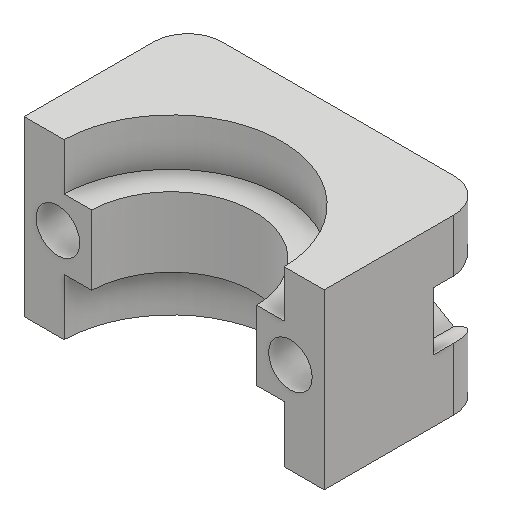
# Autodesk Inventor part: 3DP_ABS_E3DV6_Mounting_Clamp
Saved by Autodesk Inventor 2026.1 (Build 301233000, 233)
## iProperties
Created: 2016-01-19
Part Number: 3DP_ABS_E3DV6_Mounting_Clamp
Material: Ogólny
Document SubType Name: Modeling
Designer: Andrzej
Density: 1 g/cm^3
Appearance: Domyślna
Mass: 1.92147 g
Surface Area: 15.7734 cm^2
Volume: 1.92147 cm^3
Author: Andrzej
Autodesk Inventor part; units mm, degrees
ref_plane "YZ Plane" through (0, 0, 0) normal (1, 0, 0) x (0, 1, 0)
ref_plane "XZ Plane" through (0, 0, 0) normal (0, 1, 0) x (-1, 0, 0)
ref_plane "XY Plane" through (0, 0, 0) normal (0, 0, 1) x (1, 0, 0)
sketch "Szkic1" plane through (0, 0, 0) normal (0, 0, 1) x (1, 0, 0)
  line L0 (-13.054, 5.3954) -> (8.946, 5.3954)
  line L1 (8.946, 5.3954) -> (8.946, -6.6046)
  line L2 (8.946, -6.6046) -> (-13.054, -6.6046)
  line L3 (-13.054, -6.6046) -> (-13.054, 5.3954)
  point P0 (0, 0)
  dimension "d0" = 22
  dimension "d1" = 12
  constraints: 8 end point, 2 parallel, 1 horizontal, 1 perpendicular
  measures "d0" distance of L1.end L2.end
  measures "d1" distance of L0.end L1.end
extrude "Wyciągnięcie proste1" add sketch "Szkic1" along normal blind 12.7
fillet "Zaokrąglenie1" radius 2.5 2 edges at (-13.054, 5.3954, 6.35) (8.946, 5.3954, 6.35)
sketch "Szkic2" plane through (0, 0, 12.7) normal (0, 0, 1) x (1, 0, 0)
  line L0 (8.946, -6.6046) -> (8.946, 2.8954) projected
  line L1 (-13.054, 2.8954) -> (-13.054, -6.6046) projected
  circle A0 centre (-2.054, -6.8046) radius 8.075
  line L2 (6.446, 5.3954) -> (-10.554, 5.3954) projected
  point P0 (0, 0)
  dimension "d5" = 22
  dimension "d6" = 11
  dimension "d7" = 16.15
  dimension "d10" = 12.2
  constraints: 1 centre point, 1 coincident
  measures "d5" distance between parallel lines of L0 L1
  measures "d6" distance from line of L0 point (-2.054, -6.805)
  measures "d7" diameter of A0
  measures "d10" distance from line of L2 A0.centre
extrude "Wyciągnięcie proste2" cut sketch "Szkic2" against normal blind 12.7
sketch "Szkic3" plane through (0, 0, 12.7) normal (0, 0, 1) x (1, 0, 0)
  arc A0 (6.0185, -6.6046) -> (-10.1265, -6.6046) centre (-2.054, -6.8046) ccw projected
  line L0 (6.0185, -6.6046) -> (8.946, -6.6046) projected
  line L1 (8.946, -6.6046) -> (8.946, 2.8954) projected
  arc A1 (8.946, 2.8954) -> (6.446, 5.3954) centre (6.446, 2.8954) ccw projected
  line L2 (6.446, 5.3954) -> (-10.554, 5.3954) projected
  arc A2 (-10.554, 5.3954) -> (-13.054, 2.8954) centre (-10.554, 2.8954) ccw projected
  line L3 (-13.054, 2.8954) -> (-13.054, -6.6046) projected
  line L4 (-13.054, -6.6046) -> (-10.1265, -6.6046) projected
  arc A3 (3.9927, -6.6046) -> (-8.1007, -6.6046) centre (-2.054, -6.8046) ccw
  arc A4 (6.0185, -6.6046) -> (-10.1265, -6.6046) centre (-2.054, -6.8046) ccw projected
  line L5 (6.0185, -6.6046) -> (-10.1265, -6.6046)
  point P0 (0, 0)
  dimension "d11" = 12.1
  constraints: 2 end point, 2 point on circle, 2 point on line, 1 centre point, 1 coincident, 1 horizontal
  measures "d11" diameter of A3
extrude "Wyciągnięcie proste3" add sketch "Szkic3" against normal blind 8.55 contours L5 A3 A0
extrude "Wyciągnięcie proste4" cut sketch "Szkic3" against normal blind 3.45 contours L5 A3 A0
sketch "Szkic4" plane through (-13.054, -6.6046, 0) normal (0, -1, 0) x (1, 0, 0)
  line L0 (0, 0) -> (0, 12.7) projected
  line L1 (22, 0) -> (22, 12.7) projected
  line L2 (4.9533, 9.25) -> (2.9275, 9.25) projected
  line L3 (19.0725, 9.25) -> (17.0467, 9.25) projected
  line L4 (4.9533, 9.25) -> (4.9533, 4.15) projected
  line L5 (4.9533, 4.15) -> (2.9275, 4.15) projected
  point P0 (13.054, 0)
  point P1 (2.4767, 6.7)
  point P2 (19.5233, 6.7)
  dimension "d16" = 2.4766
  dimension "d17" = 2.4766
  dimension "d18" = 2.55
  dimension "d19" = 2.55
  dimension "d33" = 4.9533
  dimension "d34" = 5.1
  measures "d16" distance from line of L0 point (2.477, 6.7)
  measures "d17" distance from line of L1 point (19.523, 6.7)
  measures "d18" distance from line of L2 point (2.477, 6.7)
  measures "d19" distance from line of L3 point (19.523, 6.7)
  measures "d33" distance between parallel lines of L0 L4
  measures "d34" distance between parallel lines of L5 L2
hole "Otwór1" at (-10.5773, -6.6046, 6.7) at (6.4694, -6.6046, 6.7) direction (0, 1, 0) diameter 3.2 end through all
sketch "Szkic5" plane through (-10.554, 5.3954, 0) normal (0, 1, 0) x (1, 0, 0)
  arc A0 (0, -8.2998) -> (0, -5.1002) centre (-0.0233, -6.7) ccw projected
  line L0 (0, -12.7) -> (0, -8.2998) projected
  line L1 (17, -12.7) -> (0, -12.7) projected
  line L2 (17, -8.2998) -> (17, -12.7) projected
  arc A1 (17, -5.1002) -> (17, -8.2998) centre (17.0233, -6.7) ccw projected
  line L3 (17, 0) -> (17, -5.1002) projected
  line L4 (0, 0) -> (17, 0) projected
  line L5 (0, -5.1002) -> (0, 0) projected
  line L6 (19.5, -12.7) -> (19.5, 0) projected
  line L7 (-2.5, 0) -> (-2.5, -12.7) projected
  line L8 (-3.125, -4.9102) -> (-0.025, -3.1204)
  line L9 (-0.025, -3.1204) -> (3.075, -4.9102)
  line L10 (3.075, -4.9102) -> (3.075, -8.4898)
  line L11 (3.075, -8.4898) -> (-0.025, -10.2796)
  line L12 (-0.025, -10.2796) -> (-3.125, -8.4898)
  line L13 (-3.125, -8.4898) -> (-3.125, -4.9102)
  line L14 (13.9, -4.9102) -> (17, -3.1204)
  line L15 (17, -3.1204) -> (20.1, -4.9102)
  line L16 (20.1, -4.9102) -> (20.1, -8.4898)
  line L17 (20.1, -8.4898) -> (17, -10.2796)
  line L18 (17, -10.2796) -> (13.9, -8.4898)
  line L19 (13.9, -8.4898) -> (13.9, -4.9102)
  point P0 (10.554, 0)
  point P1 (17, -6.7)
  point P2 (-0.025, -6.7)
  point P3 (-0.025, -6.7)
  point P4 (-3.125, -6.7)
  point P5 (17, -6.7)
  point P6 (13.9, -6.7)
  constraints: 24 end point, 2 midpoint, 26 other
extrude "Wyciągnięcie proste6" cut sketch "Szkic5" against normal blind 4 contours L0 L11 L12 L7 L8 L9 L5 A0 | A0 L5 L9 L10 L11 L0 | L12 L13 L8 L7 | L18 L19 L14 L3 A1 L2 | L2 A1 L3 L15 L6 L17 | L6 L15 L16 L17
equation "\"d6\" = 0.5 * d5"
equation "\"d16\" = 0.5 * d33"
equation "\"d17\" = d16"
equation "\"d18\" = 0.5 * d34"
equation "\"d19\" = d18"
